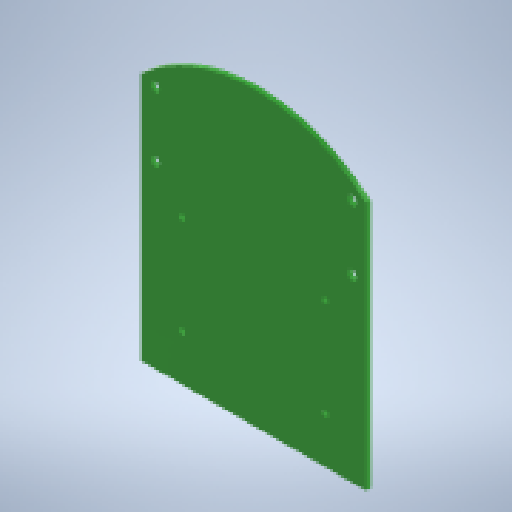
# Autodesk Inventor part: BaseBoard-SPG27
Saved by Autodesk Inventor 2025.3 (Build 293356000, 356)
## iProperties
Created: 2025-05-29
Part Number: BaseBoard-SPG27
Material: 一般
Document SubType Name: Modeling
Designer: yamashita1
Density: 1 g/cm^3
Appearance: 滑らか - 濃い深緑
CONN_W: 70.000 mm
CONN_SPAN: 23.000 mm
CONN_L1: 43.000 mm
Author: yamashita1
Autodesk Inventor part; units mm, degrees
ref_plane "YZ Plane" through (0, 0, 0) normal (1, 0, 0) x (0, 1, 0)
ref_plane "XZ Plane" through (0, 0, 0) normal (0, 1, 0) x (-1, 0, 0)
ref_plane "XY Plane" through (0, 0, 0) normal (0, 0, 1) x (1, 0, 0)
sketch "スケッチ1" plane through (0, 0, 0) normal (0, 0, 1) x (1, 0, 0)
  circle A0 centre (0, 0) radius 60 construction
  line L0 (-40, 60) -> (40, 60) construction
  line L1 (40, 60) -> (40, -60) construction
  line L2 (40, -60) -> (-40, -60) construction
  line L3 (-40, -60) -> (-40, 60) construction
  arc A1 (40, 44.7214) -> (-40, 44.7214) centre (0, 0) ccw
  line L4 (-40, 44.7214) -> (-40, -44.7214)
  line L5 (40, 44.7214) -> (40, -44.7214)
  arc A2 (-40, -44.7214) -> (40, -44.7214) centre (0, 0) ccw
  line L6 (40, -44) -> (-40, -44)
  point P0 (0, 60)
  dimension "d0" = 120
  dimension "d1" = 80
  dimension "d41" = 44
  constraints: 16 end point, 9 point on circle, 6 point on line, 3 centre point, 3 parallel, 2 perpendicular, 2 tangent, 1 coincident, 1 concentric, 1 horizontal, 1 midpoint, 1 vertical, 1 vertical alignment
  measures "d0" diameter of A0
  measures "d1" distance of L1.end L2.end
  measures "d41" distance from line of point (0, 0) L6
extrude "基板" add sketch "スケッチ1" along normal blind 1.6 contours L5 L6 L4 A1
sketch "スケッチ2" plane through (0, 0, 1.6) normal (0, 0, 1) x (1, 0, 0)
  line L0 (0, 110.7931) -> (0, -110.7931) construction
  line L1 (-40, 44.7214) -> (-40, -44) construction
  line L2 (-63.4163, -10) -> (63.4163, -10) construction
  point P0 (0, 0)
  point P1 (0, 0)
  point P2 (0, 0)
  point P3 (-42.5, -49.1808)
  point P4 (-25.5, -27.5)
  point P5 (-25.5, 7.5)
  point P6 (25.5, -27.5)
  point P7 (25.5, 7.5)
  point P8 (0, -10)
  point P9 (-40, -44)
  dimension "BLACKET_SPAN" = 35
  dimension "d40" = 10
  dimension "BLACKET_W" = 51
  constraints: 4 end point, 2 coincident, 2 horizontal alignment, 2 midpoint, 2 symmetric about line, 1 horizontal, 1 point on line, 1 vertical, 1 vertical alignment, 1 other
  measures "BLACKET_SPAN" distance of point (-25.5, 7.5) point (-25.5, -27.5)
  measures "d40" distance from line of L2 point (0, 0)
  measures "BLACKET_W" distance of point (-25.5, -27.5) point (25.5, -27.5)
hole "モータ取付穴" at (-25.5, -27.5, 1.6) at (-25.5, 7.5, 1.6) at (25.5, -27.5, 1.6) at (25.5, 7.5, 1.6) direction (0, 0, -1) diameter 2.1 end through all
sketch "スケッチ6" plane through (0, 0, 0) normal (0, 0, -1) x (-1, 0, 0)
  line L0 (0, 0) -> (0, 96.2051) construction
  point P0 (35, 43)
  point P1 (-35, 43)
  point P2 (-35, 20)
  point P3 (35, 20)
  dimension "CONN_W" = 70
  dimension "CONN_SPAN" = 23
  dimension "CONN_L1" = 43
  constraints: 2 end point, 2 symmetric about line, 1 horizontal alignment, 1 vertical, 1 vertical alignment
  measures "CONN_W" distance of point (-35, 43) point (35, 43)
  measures "CONN_SPAN" distance of point (-35, 20) point (-35, 43)
  measures "CONN_L1" vertical distance of L0.start point (35, 43)
hole "連結穴" at (-35, 43, 0) at (35, 43, 0) at (35, 20, 0) at (-35, 20, 0) direction (0, 0, 1) diameter 3.2 end through all
